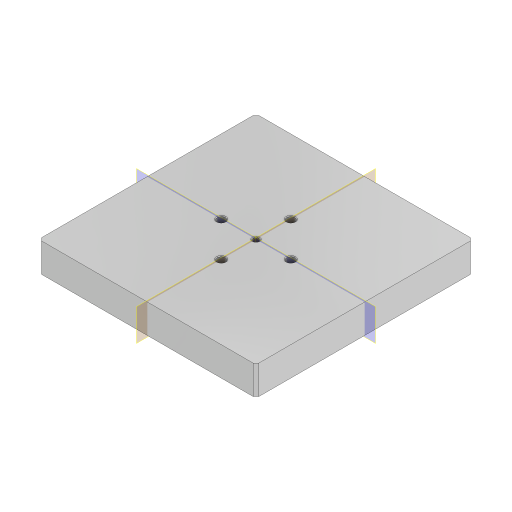
# Autodesk Inventor part: Koordinaten-Platte
Saved by Autodesk Inventor 2024.3 (Build 283343000, 343)
## iProperties
Created: 2025-05-14
Part Number: Koordinaten-Platte
Material: Generisch
Document SubType Name: Modeling
Designer: Demir
Density: 1 g/cm^3
Appearance: Aluminium - poliert
Author: Demir
Autodesk Inventor part; units mm, degrees
ref_plane "XY Plane" through (0, 0, 0) normal (0, 0, 1) x (1, 0, 0)
sketch "Skizze1" plane through (0, 0, 0) normal (0, 0, 1) x (1, 0, 0)
  line L0 (-75, 75) -> (75, 75)
  line L1 (75, 75) -> (75, -75)
  line L2 (75, -75) -> (-75, -75)
  line L3 (-75, -75) -> (-75, 75)
  line L4 (-75, 75) -> (75, -75) construction
  line L5 (75, 75) -> (-75, -75) construction
  point P0 (0, 0)
  dimension "d0" = 150
  dimension "d1" = 150
  constraints: 12 end point, 2 midpoint, 2 parallel, 1 horizontal, 1 perpendicular
  measures "d0" distance of L0.start L0.end
  measures "d1" distance of L0.end L1.end
extrude "Extrusion1" add sketch "Skizze1" along normal mid plane 20
sketch "Skizze5" plane through (0, 0, -10) normal (0, 0, -1) x (-1, 0, 0)
  line L0 (-75, -75) -> (75, -75) projected
  line L1 (75, -75) -> (75, 75) projected
  line L2 (75, 75) -> (-75, 75) projected
  line L3 (-75, 75) -> (-75, -75) projected
  circle A0 centre (0, 0) radius 13
  dimension "d30" = 26
  constraints: 1 centre point, 1 coincident
  measures "d30" diameter of A0
extrude "Extrusion3" cut sketch "Skizze5" against normal blind 6 contours A0
chamfer "Fasen2" distance 2 angle 45 4 edges at (-75, -75, 0) (75, -75, 0) (-75, 75, 0) (75, 75, 0)
chamfer "Fasen3" distance 0.5 angle 45 1 edges at (13, 0, -10)
sketch "Skizze6" plane through (0, 0, -4) normal (0, 0, -1) x (-1, 0, 0)
  circle A0 centre (0, 0) radius 13 projected
  constraints: 1 coincident
hole "Bohrung3" at (0, 0, -4) direction (0, 0, 1) diameter 4.134 end through all thread size "M5x0.8" class "6H" standard "ISO Metric profile"
sketch "Skizze7" plane through (0, 0, -10) normal (0, 0, -1) x (-1, 0, 0)
  line L0 (-75, 73) -> (-73, 75) projected
  line L1 (-75, 73) -> (-75, -73) projected
  line L2 (-73, -75) -> (-75, -73) projected
  line L3 (-73, -75) -> (73, -75) projected
  line L4 (75, -73) -> (73, -75) projected
  line L5 (75, -73) -> (75, 73) projected
  line L6 (73, 75) -> (75, 73) projected
  line L7 (73, 75) -> (-73, 75) projected
  circle A0 centre (0, 0) radius 13.5 projected
  point P0 (0, -24)
  dimension "d46" = 24
  dimension "d47" = 0
  measures "d46" distance of point (0, -24) point (0, 0)
  measures "d47" horizontal distance of point (0, 0) point (0, -24)
hole "Bohrung4" at (0, -24, -10) direction (0, 0, 1) diameter 5.5 end through all counterbore diameter 10 counterbore depth 5
pattern_circular "Runde Anordnung2" count 4 over 360 about axis through (0, 0, -10) along (0, 0, 1) of "Bohrung4"
chamfer "Fasen4" distance 0.5 angle 45 4 edges at (0, -29, -10) (29, 0, -10) (0, 29, -10) (-29, 0, -10)
chamfer "Fasen5" distance 0.5 angle 45 4 edges at (26.75, 0, 10) (0, 26.75, 10) (-26.75, 0, 10) (0, -26.75, 10)
chamfer "Fasen6" distance 0.5 angle 45 1 edges at (0, -2.067, 10)
chamfer "Fasen7" distance 0.5 angle 45 1 edges at (0, -2.067, -4)
